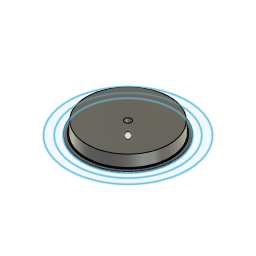
2023_04_06_CNCOrangeDigitalPringleMolding v9 (Autodesk Fusion 360 design; units mm, degrees)
Autodesk Fusion 360 part; units mm, degrees
note: some values were not read from the file. Chosen so that the rebuilt part matches the saved one: which bodies a step acts on.
sketch "Sketch1" plane through (0, 0, 0) normal (0, 0, 1) x (1, 0, 0)
  line L0 (0, 0) -> (200, 0)
  line L1 (200, 0) -> (200, 200)
  line L2 (200, 200) -> (0, 200)
  line L3 (0, 200) -> (0, 0)
  dimension "d1" = 200
  dimension "d2" = 200
  constraint horizontal L0
  constraint vertical L1
  constraint horizontal L2
  constraint vertical L3
  constraint coincident L0.start L3.end
  measures "d1" distance of L0.start L0.end
  measures "d2" distance of L0.start L2.end
extrude "Extrude1" add sketch "Sketch1" along normal blind 12 makes body 1
sketch "Sketch2" plane through (0, 0, 0) normal (0, 0, 1) x (1, 0, 0)
  circle A0 centre (50, 40) radius 38.95
  circle A1 centre (50, 40) radius 39.575
  circle A2 centre (50, 40) radius 39.325
  dimension "d5" = 77.9
  dimension "d6" = 79.15
  dimension "d15" = 78.65
  constraint concentric A0 A1
  constraint concentric A1 A2
  measures "d5" diameter of A0
  measures "d6" diameter of A1
  measures "d15" diameter of A2
extrude "Extrude2" add sketch "Sketch2" along normal blind 0.1 separate body contours A0 | A1 | A2 makes body 2
extrude "Extrude3" cut sketch "Sketch2" along normal blind 2.55 contours A1 | A2 bodies 2
extrude "Extrude5" add sketch "Sketch2" along normal blind 3.8 contours A1 | A2 bodies 2
extrude "Extrude4" cut sketch "Sketch2" along normal blind 2.55 contours A2 bodies 2 makes body 3 at (89.3783, 36.0596, 2.5333)
extrude "Extrude6" add sketch "Sketch2" along normal blind 0.1 contours A2 bodies 2 3
extrude "Extrude7" add sketch "Sketch2" along normal blind 3 separate body contours A2 makes body 4
move_body "Move1" bodies 4 to x (1, 0, 0) y (0, 1, 0) z (0, 0, 1) at (0, 0, 3.55)
combine "Combine1" operation cut target body 2 tool bodies 4
extrude "Extrude8" cut 1 faces at (88.1759, 49.7182, 3.8) along direction (0, 0, -1) blind 0.24 on bodies 2 bodies 2
extrude "Extrude9" add 1 faces at (88.1759, 49.7182, 3.56) along direction (0, 0, 1) blind 1.5 on bodies 2 bodies 2
copy_body "CopyPasteBodies1" bodies 1 makes body 5
extrude "Extrude10" cut sketch "Sketch2" along normal blind 25 contours A0 | A1 | A2 keep common part bodies 5
extrude "Extrude11" add sketch "Sketch2" along normal blind 20 separate body contours A1 | A2 makes body 6
move_body "Move2" bodies 6 to x (1, 0, 0) y (0, 1, 0) z (0, 0, 1) at (0, 0, 1.8)
combine "Combine2" operation cut target body 5 tool bodies 6
draft "Draft2" angle -4 neutral plane through (0, 0, 0) pull (0, 0, -1) 1 faces at (88.7564, 43.8782, 8.6) on bodies 5
sketch "AirHole" plane through (0, 0, 0) normal (0, 0, 1) x (1, 0, 0)
  circle A0 centre (50, 40) radius 3
  circle A1 centre (50, 40) radius 0.5
  dimension "d28" = 6
  dimension "d29" = 1
  constraint concentric A0 A1
  measures "d28" diameter of A0
  measures "d29" diameter of A1
extrude "Extrude12" cut sketch "AirHole" along normal blind 26 contours A0 | A1 bodies 5
sketch "Sketch4" plane through (0, 0, 0) normal (0, 0, 1) x (1, 0, 0)
  circle A0 centre (50, 40) radius 42.1814
extrude "Extrude13" add sketch "Sketch4" along normal blind 1 bodies 5
extrude "Extrude14" cut sketch "AirHole" along normal blind 15 contours A0 | A1 bodies 5
sketch "Sketch5" plane through (0, 0, 0) normal (1, 0, 0) x (0, 1, 0)
sketch "Sketch6" plane through (0, 0, 0) normal (1, 0, 0) x (0, 1, 0)
sketch "Sketch7" plane through (0, 0, 0) normal (0, 0, 1) x (1, 0, 0)
  circle A0 centre (50, 40) radius 42.2
  circle A1 centre (50, 40) radius 42.2
  circle A2 centre (50, 40) radius 48.2
  circle A3 centre (50, 40) radius 55.2268
  dimension "d41" = 84.4
  dimension "d42" = 96.4
  constraint concentric A0 A1
  constraint concentric A1 A2
  constraint concentric A2 A3
  measures "d41" diameter of A1
  measures "d42" diameter of A2
extrude "Extrude15" add sketch "Sketch7" along normal blind 12 separate body contours A3 makes body 7
hidden bodies 1 2 7
equation "d3 = WoodHeight"
equation "d5 = d6 - 1.25 mm"
equation "d15 = d6 - 0.5 mm"
equation "WoodHeight = 12 mm"
equation "d42 = d41 + 12 mm"
equation "CutDim = 6 mm"
equation "d44 = WoodHeight"
named bodies: "Wood Original", "Pringle Top", "Wood Original (1)"
